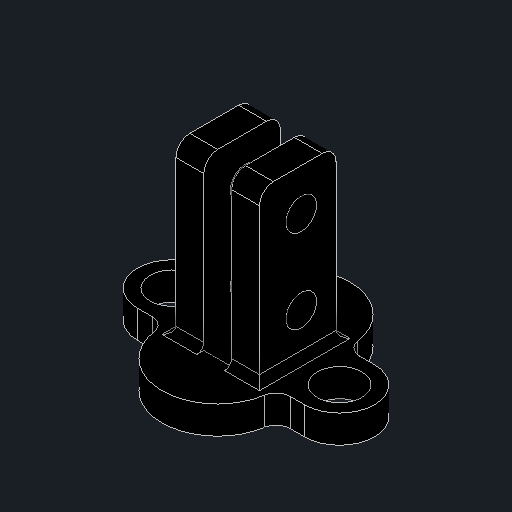
# Autodesk Inventor part: CarbonConnectorStabPCBConnector
Saved by Autodesk Inventor 2023 (Build 270158000, 158)
## iProperties
Created: 2023-02-24
Part Number: CarbonConnectorStabPCBConnector
Material: Generic
Document SubType Name: Modeling
Designer: Elias Braun
Density: 1 g/cm^3
Appearance: Default
Author: Elias Braun
Autodesk Inventor part; units mm, degrees
ref_plane "YZ Plane" through (0, 0, 0) normal (1, 0, 0) x (0, 1, 0)
ref_plane "XZ Plane" through (0, 0, 0) normal (0, 1, 0) x (-1, 0, 0)
ref_plane "XY Plane" through (0, 0, 0) normal (0, 0, 1) x (1, 0, 0)
sketch "Sketch1" plane through (0, 0, 0) normal (0, 1, 0) x (-1, 0, 0)
  circle A0 centre (6, 0) radius 1.6
  circle A1 centre (6, 0) radius 1.6
  circle A2 centre (-6, 0) radius 1.6
  circle A3 centre (-6, 0) radius 1.6
  line L0 (1, 2.75) -> (1, -2.75) construction
  line L1 (1, 2.75) -> (-1, 2.75)
  line L2 (-1, -2.75) -> (-1, 2.75) construction
  line L3 (-1, -2.75) -> (1, -2.75)
  line L4 (0, 2.75) -> (0, -2.75) construction
  line L5 (-1, -2.75) -> (-3, -2.75)
  line L6 (-3, -2.75) -> (-3, 2.75)
  line L7 (-3, 2.75) -> (-1, 2.75)
  line L8 (-1, 2.75) -> (-1, -2.75)
  line L9 (1, -2.75) -> (3, -2.75)
  line L10 (3, -2.75) -> (3, 2.75)
  line L11 (3, 2.75) -> (1, 2.75)
  line L12 (1, 2.75) -> (1, -2.75)
  line L13 (6, 0) -> (-6, 0) construction
  arc A4 (6, -2.5) -> (6, 2.5) centre (6, 0) ccw
  arc A5 (-6, 2.5) -> (-6, -2.5) centre (-6, 0) ccw
  line L14 (0, 2.75) -> (0, -2.75) construction
  arc A6 (4, 2.75) -> (-4, 2.75) centre (0, 2.75) ccw
  arc A7 (-4, -2.75) -> (4, -2.75) centre (0, -2.75) ccw
  line L15 (4, -2.75) -> (4, -2.5)
  line L16 (4, 2.5) -> (4, 2.75)
  line L17 (-4, 2.75) -> (-4, 2.5)
  line L18 (-4, -2.5) -> (-4, -2.75)
  line L19 (-6, -2.5) -> (-4, -2.5)
  line L20 (4, -2.5) -> (6, -2.5)
  line L21 (6, 2.5) -> (4, 2.5)
  line L22 (-4, 2.5) -> (-6, 2.5)
  point P0 (0, 0)
  point P1 (0, 0)
  point P2 (0, 0)
  point P3 (0, 0)
  point P4 (0, 0)
  point P5 (0, 0)
  dimension "d6" = 2
  dimension "d7" = 2
  dimension "d8" = 5
  dimension "d9" = 8
  constraints: 52 end point, 16 tangent, 13 equal length, 8 centre point, 8 point on circle, 5 midpoint, 3 horizontal, 2 coincident, 2 perpendicular, 1 point on line
  measures "d6" distance of L6.end L7.end
  measures "d7" distance of L11.end L10.end
  measures "d8" diameter of A5
  measures "d9" diameter of A7
extrude "Extrusion1" add sketch "Sketch1" along normal blind 2 contours L11 L10 L9 L12 | L8 L5 L6 L7 | L20 L15 A7 L18 L19 A5 L22 L17 A6 L16 L21 A4
fillet "Fillet1" radius 1 4 edges at (4, 1, -2.5) (4, 1, 2.5) (-4, 1, -2.5) (-4, 1, 2.5)
sketch "Sketch3" plane through (0, 2, 0) normal (0, 1, 0) x (1, 0, 0)
  line L0 (1, -2.75) -> (-1, -2.75) projected
  line L1 (1, -2.75) -> (3, -2.75)
  line L2 (3, -2.75) -> (3, 2.75)
  line L3 (3, 2.75) -> (1, 2.75)
  line L4 (1, 2.75) -> (1, -2.75)
  line L5 (-1, -2.75) -> (-3, -2.75)
  line L6 (-3, -2.75) -> (-3, 2.75)
  line L7 (-3, 2.75) -> (-1, 2.75)
  line L8 (-1, 2.75) -> (-1, -2.75)
  point P0 (0, 0)
  dimension "d11" = 2
  dimension "d12" = 5.5
  dimension "d13" = 2
  constraints: 16 end point, 4 parallel, 2 horizontal, 2 perpendicular, 1 point on line
  measures "d11" distance of L3.end L2.end
  measures "d12" distance of L2.end L1.end
  measures "d13" distance of L6.end L7.end
extrude "Extrusion2" add sketch "Sketch3" along normal blind 12
fillet "Fillet2" radius 0.5 6 edges at (2, 2, -2.75) (-2, 2, -2.75) (-3, 2, 0) (3, 2, 0) (2, 2, 2.75) (-2, 2, 2.75)
sketch "Sketch4" plane through (3, 14, 2.75) normal (1, 0, 0) x (0, 0, -1)
  line L0 (5.5, 0) -> (0.5, 0) construction
  line L1 (5.5, -12) -> (5.5, 0) construction
  line L2 (0.5, 0) -> (5.5, -12) construction
  line L3 (3, -6) -> (3, -9) construction
  line L4 (3, -6) -> (3.9934, -6) construction
  circle A0 centre (3, -9) radius 1.1
  circle A1 centre (3, -3) radius 1.1
  line L5 (0, 0) -> (5.5, 0) projected
  point P0 (2.75, -14)
  point P1 (52.5, -13.5)
  dimension "d17" = 3
  dimension "d18" = 2.2
  constraints: 10 end point, 2 centre point, 1 coincident, 1 horizontal, 1 midpoint, 1 symmetric about line, 1 vertical, 1 other
  measures "d17" distance of L3.start L3.end
  measures "d18" diameter of A0
extrude "Extrusion3" cut sketch "Sketch4" against normal blind 12
fillet "Fillet3" radius 1 4 edges at (2, 14, -2.75) (-2, 14, -2.75) (2, 14, 2.75) (-2, 14, 2.75)
body "Solid1"
